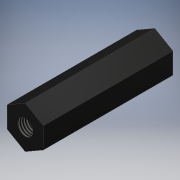
# Autodesk Inventor part: Entretoise25mm
Saved by Autodesk Inventor 2019 (Build 230136000, 136)
## iProperties
Created: 2019-07-30
Part Number: Entretoise25mm
Material: Plastique ABS
Document SubType Name: Modeling
Designer: Sébastien DI MERCURIO
Mass: 0.937217 g
Surface Area: 9.12571 cm^2
Volume: 0.884167 cm^3
Density: 1.06 g/cm^3
Appearance: Lustré - Noir
Author: Sébastien DI MERCURIO
Autodesk Inventor part; units mm, degrees
ref_plane "YZ Plane" through (0, 0, 0) normal (1, 0, 0) x (0, 1, 0)
ref_plane "XZ Plane" through (0, 0, 0) normal (0, 1, 0) x (-1, 0, 0)
ref_plane "XY Plane" through (0, 0, 0) normal (0, 0, 1) x (1, 0, 0)
sketch "Esquisse1" plane through (0, 0, 0) normal (0, 0, 1) x (1, 0, 0)
  line L0 (0, 4.0415) -> (3.5, 2.0207)
  line L1 (3.5, 2.0207) -> (3.5, -2.0207)
  line L2 (3.5, -2.0207) -> (0, -4.0415)
  line L3 (0, -4.0415) -> (-3.5, -2.0207)
  line L4 (-3.5, -2.0207) -> (-3.5, 2.0207)
  line L5 (-3.5, 2.0207) -> (0, 4.0415)
  circle A0 centre (0, 0) radius 1.5
  dimension "d0" = 3
  dimension "d1" = 7
  constraints: 12 end point, 2 coincident, 1 centre point, 1 vertical alignment, 13 other
  measures "d0" diameter of A0
  measures "d1" distance between parallel lines of L3 L0
extrude "Extrusion1" add sketch "Esquisse1" along normal blind 25
thread "Filetage1" size "M3x0.5" class "6H" standard "ANSI Metric M Profile" full length
